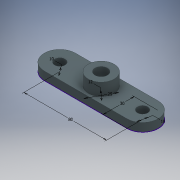
# Autodesk Inventor part: lab3_1
Saved by Autodesk Inventor 2018 (Build 220112000, 112)
## iProperties
Created: 2020-04-08
Part Number: lab3_1
Material: Свинец
Document SubType Name: Modeling
Designer: Antony
Density: 11.34 g/cm^3
Appearance: Свинец
Author: Antony
Autodesk Inventor part; units mm, degrees
ref_plane "YZ Plane" through (0, 0, 0) normal (1, 0, 0) x (0, 1, 0)
ref_plane "XZ Plane" through (0, 0, 0) normal (0, 1, 0) x (-1, 0, 0)
ref_plane "XY Plane" through (0, 0, 0) normal (0, 0, 1) x (1, 0, 0)
sketch "Эскиз1" plane through (0, 0, 0) normal (0, 0, 1) x (1, 0, 0)
  line L0 (-40, 0) -> (40, 0) construction
  line L1 (-40, -15) -> (40, -15)
  line L2 (40, 15) -> (-40, 15)
  arc A0 (-40, 15) -> (-40, -15) centre (-40, 0) ccw
  arc A1 (40, -15) -> (40, 15) centre (40, 0) ccw
  circle A2 centre (0, 0) radius 12.5
  circle A3 centre (0, 0) radius 6
  circle A4 centre (40, 0) radius 5
  circle A5 centre (-40, 0) radius 5
  dimension "d2" = 80
  dimension "d3" = 30
  dimension "d4" = 25
  dimension "d5" = 12
  dimension "d6" = 10
  dimension "d7" = 10
  constraints: 8 end point, 6 centre point, 4 coincident, 4 point on circle, 4 tangent, 1 horizontal, 1 midpoint, 1 parallel
  measures "d2" distance of L0.end L0.start
  measures "d3" distance of L1.end L2.start
  measures "d4" diameter of A2
  measures "d5" diameter of A3
  measures "d6" diameter of A4
  measures "d7" diameter of A5
extrude "Выдавливание1" add sketch "Эскиз1" along normal blind 8 contours A0 L2 A1 L1 | A2 | A4 | A5
extrude "Выдавливание2" cut sketch "Эскиз1" along normal blind 8 contours A4 | A5
extrude "Выдавливание3" add sketch "Эскиз1" along normal blind 20 contours A2
